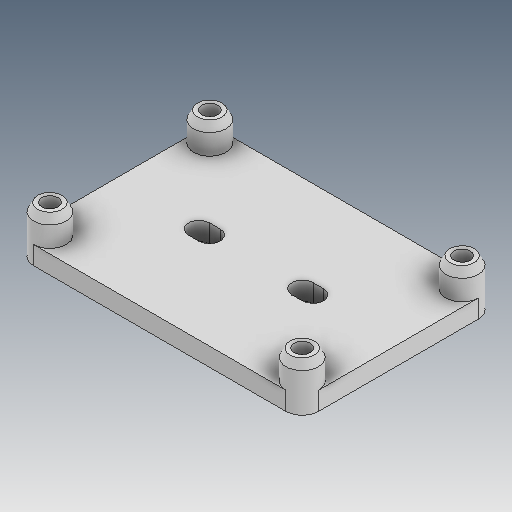
# Autodesk Inventor part: proto-board_standoffs_plate
Saved by Autodesk Inventor 2025.1 (Build 291241000, 241)
## iProperties
Created: 2026-07-06
Part Number: proto-board_standoffs_plate
Material: Generic
Document SubType Name: Modeling
Designer: Aiden
Density: 1 g/cm^3
Appearance: Default
Author: Aiden
Autodesk Inventor part; units mm, degrees
ref_plane "YZ Plane" through (0, 0, 0) normal (1, 0, 0) x (0, 1, 0)
ref_plane "XZ Plane" through (0, 0, 0) normal (0, 1, 0) x (-1, 0, 0)
ref_plane "XY Plane" through (0, 0, 0) normal (0, 0, 1) x (1, 0, 0)
sketch "proto-board hole layout" plane through (0, 0, 0) normal (0, 1, 0) x (-1, 0, 0)
  circle A0 centre (6.6395, -4.3647) radius 1.49
  circle A1 centre (-55.3405, -4.3647) radius 1.49
  circle A2 centre (-55.3405, 34.9153) radius 1.49
  circle A3 centre (6.6395, 34.9153) radius 1.49
  line L0 (5.1495, -4.3647) -> (-53.8505, -4.3647) construction
  line L1 (5.1495, 34.9153) -> (-53.8505, 34.9153) construction
  line L2 (-55.3405, 33.4253) -> (-55.3405, -2.8747) construction
  line L3 (6.6395, 33.4253) -> (6.6395, -2.8747) construction
  dimension "d0" = 2.98
  dimension "d1" = 59
  dimension "d2" = 36.3
  constraints: 8 end point, 8 point on circle, 4 centre point, 4 coincident, 3 equal radius, 2 horizontal alignment, 2 parallel, 2 vertical alignment, 1 horizontal, 1 perpendicular
  measures "d0" diameter of A0
  measures "d1" distance of L0.start L0.end
  measures "d2" distance of L3.start L3.end
sketch "Sketch3" plane through (0, 0, 0) normal (0, 1, 0) x (-1, 0, 0)
  circle A0 centre (6.6395, -4.3647) radius 1.49 projected
  circle A1 centre (6.6395, -4.3647) radius 4
  point P0 (0, 0)
  dimension "d15" = 8
  constraints: 1 centre point, 1 coincident
  measures "d15" diameter of A1
extrude "Extrusion2" add sketch "Sketch3" along normal blind 7 contours A0 | A1
sketch "Sketch4" plane through (-6.6395, 7, -4.3647) normal (0, 1, 0) x (1, 0, 0)
  circle A0 centre (0, 0) radius 4 construction
  point P0 (6.6395, -4.3647)
  constraints: 1 coincident
hole "Hole1" at (-6.6395, 7, -4.3647) direction (0, -1, 0) diameter 4 depth 5 tip angle 118
chamfer "Chamfer1" distance 1 distance2 2 1 edges at (-2.6395, 7, -4.3647) measured on face at (-3.1395, 7, -4.3647)
pattern_sketch "Sketch Driven Pattern1" from (-6.6395, 0, -4.3647) copies at (55.3405, 0, -4.3647) at (55.3405, 0, 34.9153) at (-6.6395, 0, 34.9153)
sketch "Sketch5" plane through (-6.6395, 0, 34.9153) normal (0, -1, 0) x (1, 0, 0)
  circle A0 centre (0, 0) radius 4 projected
  circle A1 centre (61.98, 0) radius 4 projected
  circle A2 centre (61.98, -39.28) radius 4 projected
  circle A3 centre (0, -39.28) radius 4 projected
  line L0 (-4, 4) -> (65.98, 4)
  line L1 (65.98, 4) -> (65.98, -43.28)
  line L2 (65.98, -43.28) -> (-4, -43.28)
  line L3 (-4, -43.28) -> (-4, 4)
  point P0 (6.6395, -34.9153)
  point P1 (-4, 0)
  point P2 (-4, -39.28)
  point P3 (0, -43.28)
  point P4 (61.98, -43.28)
  point P5 (65.98, -39.28)
  point P6 (65.98, 0)
  point P7 (61.98, 4)
  point P8 (0, 4)
  constraints: 8 end point, 5 tangent, 2 parallel, 1 horizontal, 1 perpendicular
extrude "Extrusion3" add sketch "Sketch5" along normal blind 4.5 contours A0 | A0 L0 A1 L1 A2 L2 A3 L3 | A1 | A3 | A2
sketch "Sketch6" plane through (-6.6395, 0, 34.9153) normal (0, 1, 0) x (1, 0, 0)
  line L0 (0, 43.28) -> (61.98, 43.28) projected
  line L1 (30.99, 43.28) -> (30.99, -4) construction
  line L2 (61.98, -4) -> (0, -4) projected
  line L3 (-4, 0) -> (-4, 39.28) projected
  line L4 (-4, 19.64) -> (65.98, 19.64) construction
  line L5 (65.98, 39.28) -> (65.98, 0) projected
  line L6 (19.56, 19.64) -> (17.02, 19.64) construction
  line L7 (19.56, 17.04) -> (17.02, 17.04)
  line L8 (17.02, 22.24) -> (19.56, 22.24)
  arc A0 (19.56, 17.04) -> (19.56, 22.24) centre (19.56, 19.64) ccw
  arc A1 (17.02, 22.24) -> (17.02, 17.04) centre (17.02, 19.64) ccw
  line L9 (42.42, 17.04) -> (44.96, 17.04)
  line L10 (44.96, 22.24) -> (42.42, 22.24)
  arc A2 (42.42, 22.24) -> (42.42, 17.04) centre (42.42, 19.64) ccw
  arc A3 (44.96, 17.04) -> (44.96, 22.24) centre (44.96, 19.64) ccw
  point P0 (6.6395, 34.9153)
  point P1 (18.29, 19.64)
  point P2 (18.29, 22.24)
  point P3 (18.29, 17.04)
  dimension "d21" = 11.43
  dimension "d22" = 13.97
  dimension "d23" = 5.2
  constraints: 16 end point, 8 point on circle, 7 midpoint, 6 symmetric about line, 4 centre point, 4 tangent, 2 point on line, 1 collinear, 1 parallel, 2 other
  measures "d21" distance from line of L1 L6.start
  measures "d22" distance from line of L1 L6.end
  measures "d23" distance of point (18.29, 22.24) point (18.29, 17.04)
extrude "Extrusion4" cut sketch "Sketch6" against normal blind 4.5
body "Solid2"
